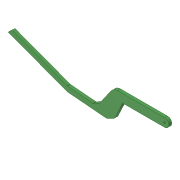
# Autodesk Inventor part: Kermit Mount
Saved by Autodesk Inventor 2018.2 (Build 222227000, 227)
## iProperties
Created: 2018-03-05
Part Number: Kermit Mount
Material: Generic
Document SubType Name: Modeling
Designer: lopez.xavier
Density: 1 g/cm^3
Appearance: Smooth - Dark Forest Green
Mass: 1210.68 g
Surface Area: 1699.27 cm^2
Volume: 1210.68 cm^3
Author: lopez.xavier
Autodesk Inventor part; units mm, degrees
ref_plane "YZ Plane" through (0, 0, 0) normal (1, 0, 0) x (0, 1, 0)
ref_plane "XZ Plane" through (0, 0, 0) normal (0, 1, 0) x (-1, 0, 0)
ref_plane "XY Plane" through (0, 0, 0) normal (0, 0, 1) x (1, 0, 0)
sketch "Sketch1" plane through (0, 0, 0) normal (0, 0, 1) x (1, 0, 0)
  line L0 (0, 0) -> (1104.9, 0)
  line L1 (1104.9, 0) -> (1104.9, 203.2)
  line L2 (1104.9, 203.2) -> (0, 203.2)
  line L3 (0, 203.2) -> (0, 0)
  dimension "d0" = 1104.9
  dimension "d1" = 203.2
  constraints: 8 end point, 2 parallel, 1 horizontal, 1 perpendicular
  measures "d0" distance of L1.end L2.end
  measures "d1" distance of L0.end L1.end
extrude "Extrusion1" add sketch "Sketch1" along normal blind 20.32
sketch "Sketch2" plane through (0, 0, 20.32) normal (0, 0, 1) x (1, 0, 0)
  line L0 (1104.9, 0) -> (1104.9, 203.2) projected
  line L1 (0, 0) -> (1104.9, 0) projected
  line L2 (1104.9, 57.15) -> (723.9, 57.15)
  line L3 (723.9, 57.15) -> (723.9, 0)
  line L4 (723.9, 0) -> (1104.9, 0)
  line L5 (1104.9, 0) -> (1104.9, 57.15)
  line L6 (723.9, 0) -> (629.2025, 135.242)
  line L7 (723.9, 0) -> (671.9967, -36.3431)
  line L8 (629.2025, 135.242) -> (585.2084, 160.642)
  line L9 (585.2084, 160.642) -> (407.4084, 145.0865)
  line L10 (787.4, 57.15) -> (731.14, 177.8)
  line L11 (731.14, 177.8) -> (676.6695, 203.2)
  line L12 (1104.9, 203.2) -> (0, 203.2) projected
  line L13 (676.6695, 203.2) -> (407.4084, 179.6427)
  line L14 (787.4, 57.15) -> (723.9, 57.15)
  line L15 (723.9, 57.15) -> (723.9, 0)
  line L16 (407.4084, 179.6427) -> (0, 27.5632)
  line L17 (407.4084, 145.0865) -> (26.4084, 2.8648)
  line L18 (0, 203.2) -> (0, 0) projected
  line L19 (26.4084, 2.8648) -> (0, 27.5632)
  line L20 (407.4084, 145.0865) -> (365.4136, 141.4124)
  dimension "d4" = 57.15
  dimension "d5" = 381
  dimension "d6" = 125
  dimension "d7" = 165.1
  dimension "d8" = 50.8
  dimension "d9" = 155
  dimension "d10" = 145
  dimension "d11" = 177.8
  dimension "d12" = 317.5
  dimension "d13" = 115
  dimension "d14" = 120.65
  dimension "d15" = 140
  dimension "d16" = 0
  dimension "d18" = 381
  dimension "d19" = 0
  dimension "d33" = 15.47
  constraints: 34 end point, 4 parallel, 4 point on line, 3 perpendicular, 2 collinear, 1 horizontal
  measures "d4" distance of L2.end L3.end
  measures "d5" distance of L2.start L2.end
  measures "d6" angle of L1 L6
  measures "d7" distance from line of L6.end L7
  measures "d8" distance of L6.end L8.end
  measures "d9" angle of L6 L8
  measures "d10" angle of L8 L9
  measures "d11" horizontal distance of L8.end L9.end
  measures "d12" distance from line of L0 L10.start
  measures "d13" angle of L2 L10
  measures "d14" vertical distance of L10.start L10.end
  measures "d15" angle of L10 L11
  measures "d16" horizontal distance of L9.end L13.end
  measures "d18" horizontal distance of L9.end L17.end
  measures "d19" distance from line of L18 L16.end
  measures "d33" angle of L17 L20
extrude "Extrusion2" cut sketch "Sketch2" against normal blind 20.32 contours L2 L10 L11 L12 L0 | L1 L18 L19 L17 L9 L8 L6 | L13 L16 L18 L12
fillet "Fillet1" radius 28.575 2 edges at (1104.9, 0, 10.16) (1104.9, 57.15, 10.16)
fillet "Fillet2" radius 57.15 1 edges at (723.9, 0, 10.16)
fillet "Fillet3" radius 6.35 3 edges at (629.2025, 135.242, 10.16) (585.2084, 160.642, 10.16) (407.4084, 145.0865, 10.16)
fillet "Fillet4" radius 25.4 3 edges at (676.6695, 203.2, 10.16) (731.14, 177.8, 10.16) (407.4084, 179.6427, 10.16)
sketch "Sketch3" plane through (0, 0, 0) normal (0, 0, -1) x (-1, 0, 0)
  circle A0 centre (-1076.325, 28.575) radius 6.35
  line L0 (-753.6504, 0) -> (-1076.325, 0) projected
  arc A1 (-1076.325, 57.15) -> (-1076.325, 0) centre (-1076.325, 28.575) ccw projected
  point P0 (0, 0)
  dimension "d26" = 12.7
  dimension "d29" = 0
  dimension "d30" = 0
  constraints: 1 centre point
  measures "d26" diameter of A0
  measures "d29" distance of A1.centre A0.centre
  measures "d30" distance of A1.centre A0.centre
extrude "Extrusion3" cut sketch "Sketch3" against normal blind 20.32
body "Solid1"
